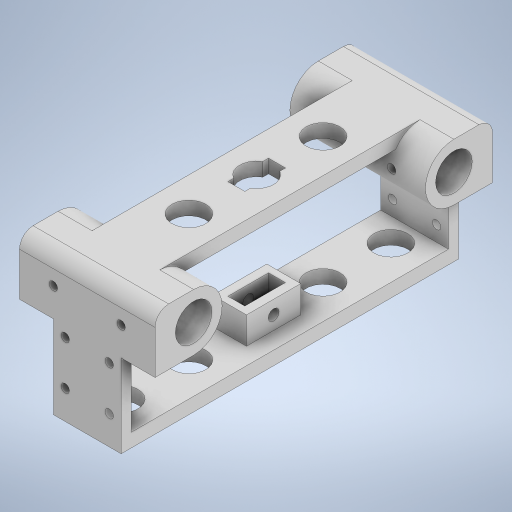
# Autodesk Inventor part: top
Saved by Autodesk Inventor 2024 (Build 280153000, 153)
## iProperties
Created: 2024-07-02
Part Number: top
Material: 일반
Document SubType Name: Modeling
Designer: Gihyeok Na
Density: 1 g/cm^3
Appearance: 기본값
Author: Gihyeok Na
Autodesk Inventor part; units mm, degrees
ref_plane "YZ Plane" through (0, 0, 0) normal (1, 0, 0) x (0, 1, 0)
ref_plane "XZ Plane" through (0, 0, 0) normal (0, 1, 0) x (-1, 0, 0)
ref_plane "XY Plane" through (0, 0, 0) normal (0, 0, 1) x (1, 0, 0)
sketch "스케치1" plane through (0, 0, 0) normal (1, 0, 0) x (0, 1, 0)
  line L0 (-15, -8.4) -> (15, -8.4)
  line L1 (15, -8.4) -> (15, -11.4)
  line L2 (15, -11.4) -> (-15, -11.4)
  line L3 (-15, -11.4) -> (-15, -8.4)
  line L4 (-15, -8.4) -> (15, -11.4) construction
  line L5 (15, -8.4) -> (-15, -11.4) construction
  line L6 (-10.7716, 0) -> (20.6854, 0) construction
  circle A0 centre (17.9, 0) radius 5.4
  circle A1 centre (17.9, 0) radius 8.4
  line L7 (9.5, -4.3302) -> (9.5, -23.7251) construction
  line L8 (15, -8.4) -> (17.9, -8.4)
  line L9 (9.5, 0) -> (9.5, -8.4)
  line L10 (56.0253, 38.4) -> (-49.003, 38.4) construction
  line L11 (-15, 85.2) -> (15, 85.2)
  line L12 (15, 85.2) -> (15, 88.2)
  line L13 (15, 88.2) -> (-15, 88.2)
  line L14 (-15, 88.2) -> (-15, 85.2)
  line L15 (-15, 85.2) -> (15, 88.2) construction
  line L16 (15, 85.2) -> (-15, 88.2) construction
  line L17 (-10.7716, 76.8) -> (20.6854, 76.8) construction
  circle A2 centre (17.9, 76.8) radius 5.4
  circle A3 centre (17.9, 76.8) radius 8.4
  line L18 (9.5, 81.1302) -> (9.5, 100.5251) construction
  line L19 (15, 85.2) -> (17.9, 85.2)
  line L20 (9.5, 76.8) -> (9.5, 85.2)
  line L21 (15, -11.4) -> (26.3, -11.4)
  line L22 (26.3, -11.4) -> (26.3, 0)
  line L23 (15, 88.2) -> (26.3, 88.2)
  line L24 (26.3, 88.2) -> (26.3, 76.8)
  point P0 (0, -9.9)
  point P1 (6.5, -8.4)
  point P2 (22.1201, -7.263)
  point P3 (0, 86.7)
  point P4 (6.5, 85.2)
  point P5 (22.1201, 84.063)
  dimension "d2" = 30
  dimension "d3" = 3
  dimension "d9" = 10.8
  dimension "d10" = 16.8
  dimension "d11" = 8.5
  dimension "d12" = 3
  dimension "d20" = 38.4
  constraints: 50 end point, 18 symmetric about line, 11 point on line, 7 point on circle, 4 centre point, 4 horizontal, 4 midpoint, 3 tangent, 2 coincident, 2 parallel, 1 perpendicular, 1 vertical, 2 other
  measures "d2" distance of L0.start L0.end
  measures "d3" distance of L0.end L1.end
  measures "d9" diameter of A0
  measures "d10" diameter of A1
  measures "d11" distance from line of point (6.5, -8.4) L1
  measures "d12" distance from line of L7 point (6.5, -8.4)
  measures "d20" distance from line of L10 A0.centre
extrude "돌출1" add sketch "스케치1" along normal mid plane 20
fillet "모깎기1" radius 4 2 edges at (0, 26.3, -11.4) (0, 26.3, 88.2)
sketch "스케치4" plane through (10, -15, -11.4) normal (0, 0, -1) x (-1, 0, 0)
  line L0 (-6.6272, 15) -> (50.9826, 15) construction
  line L1 (10, 54.1091) -> (10, -11.8144) construction
  circle A0 centre (3.5, 8.5) radius 1.25
  line L2 (20, 0) -> (0, 0) projected
  line L3 (0, 0) -> (0, 37.3) projected
  circle A1 centre (16.5, 8.5) radius 1.25
  circle A2 centre (3.5, 21.5) radius 1.25
  circle A3 centre (16.5, 21.5) radius 1.25
  circle A4 centre (10, 32.9) radius 1.25
  line L4 (20, 41.3) -> (0, 41.3) projected
  point P0 (10, 15)
  dimension "d22" = 2.5
  dimension "d23" = 8.5
  dimension "d24" = 3.5
  dimension "d27" = 2.5
  dimension "d28" = 8.4
  constraints: 5 centre point, 4 end point, 3 symmetric about line, 1 horizontal, 1 point on line, 1 vertical, 3 other
  measures "d22" diameter of A0
  measures "d23" distance from line of L2 A0.centre
  measures "d24" distance from line of L3 A0.centre
  measures "d27" diameter of A4
  measures "d28" distance from line of A4.centre L4
extrude "돌출4" cut sketch "스케치4" against normal through all contours A0 | A1 | A2 | A3
sketch "스케치5" plane through (-10, 0, 0) normal (-1, 0, 0) x (0, 0, 1)
  circle A0 centre (0, 17.9) radius 5.4 projected
  arc A1 (-7.4, 26.3) -> (-11.4, 22.3) centre (-7.4, 22.3) ccw projected
  line L0 (-11.4, 22.3) -> (-11.4, -15) projected
  line L1 (-11.4, -15) -> (-8.4, -15) projected
  line L2 (-8.4, -15) -> (-8.4, 9.5) projected
  line L3 (-8.4, 9.5) -> (0, 9.5) projected
  arc A2 (0, 9.5) -> (0, 26.3) centre (0, 17.9) ccw projected
  line L4 (0, 26.3) -> (-7.4, 26.3) projected
  circle A3 centre (76.8, 17.9) radius 5.4 projected
  arc A4 (88.2, 22.3) -> (84.2, 26.3) centre (84.2, 22.3) ccw projected
  line L5 (84.2, 26.3) -> (76.8, 26.3) projected
  arc A5 (76.8, 26.3) -> (76.8, 9.5) centre (76.8, 17.9) ccw projected
  line L6 (76.8, 9.5) -> (85.2, 9.5) projected
  line L7 (85.2, 9.5) -> (85.2, -15) projected
  line L8 (85.2, -15) -> (88.2, -15) projected
  line L9 (88.2, -15) -> (88.2, 22.3) projected
  line L10 (-8.4, -15) -> (85.2, -15)
  line L11 (-8.4, -11) -> (85.2, -11)
  line L12 (85.2, -15) -> (88.2, -15) projected
  line L13 (-8.4, 9.5) -> (-8.4, -15) projected
  line L14 (0, 26.3) -> (76.8, 26.3)
  circle A6 centre (0, 17.9) radius 5.4 projected
  circle A7 centre (76.8, 17.9) radius 5.4 projected
  line L15 (7.1554, 22.3) -> (69.6446, 22.3)
  point P0 (0, 0)
  point P1 (0, -6.5)
  point P2 (0, 6.5)
  point P3 (0, 0)
  point P4 (85.2, -4.062)
  dimension "d29" = 4
  dimension "d31" = 8.5
  dimension "d32" = 13
  dimension "d35" = 4
  constraints: 8 end point, 3 horizontal, 3 point on line, 2 point on circle, 2 tangent, 1 collinear, 1 perpendicular
  measures "d29" distance between parallel lines of L10 L11
  measures "d31" distance from line of L10 point (0, -6.5)
  measures "d32" distance of point (0, -6.5) point (0, 6.5)
  measures "d35" distance between parallel lines of L15 L14
extrude "돌출5" add sketch "스케치5" against normal up to surface (20 mm away) contours L14 A5 L15 A2 | L2 L11 L7 L10
sketch "스케치6" plane through (-10, -15, -11.4) normal (0, -1, 0) x (1, 0, 0)
  circle A0 centre (10, 10) radius 5
  line L0 (0, 0) -> (20, 0) projected
  line L1 (10, 10) -> (10, 54.4458) construction
  circle A1 centre (10, 89.6) radius 5
  line L2 (0, 99.6) -> (20, 99.6) projected
  circle A2 centre (10, 30) radius 5
  circle A3 centre (10, 69.6) radius 5
  circle A4 centre (10, 49.6) radius 5
  line L3 (7.5, 55.6) -> (7.5, 43.6)
  line L4 (7.5, 43.6) -> (12.5, 43.6)
  line L5 (12.5, 43.6) -> (12.5, 55.6)
  line L6 (12.5, 55.6) -> (7.5, 55.6)
  line L7 (7.5, 55.6) -> (12.5, 43.6) construction
  line L8 (7.5, 43.6) -> (12.5, 55.6) construction
  line L9 (5, 57.6) -> (5, 41.6)
  line L10 (5, 41.6) -> (15, 41.6)
  line L11 (15, 41.6) -> (15, 57.6)
  line L12 (15, 57.6) -> (5, 57.6)
  line L13 (5, 57.6) -> (15, 41.6) construction
  line L14 (5, 41.6) -> (15, 57.6) construction
  line L15 (20, 55.6) -> (0, 55.6)
  line L16 (0, 96.6) -> (0, 3) projected
  line L17 (20, 43.6) -> (0, 43.6)
  line L18 (20, 99.6) -> (20, 0) projected
  line L19 (0, 0) -> (0, 99.6) projected
  point P0 (10, 11.4)
  point P1 (7.5, 53.9301)
  point P2 (12.5, 53.9301)
  point P3 (12.5, 45.2699)
  point P4 (7.5, 45.2699)
  dimension "d38" = 10
  dimension "d39" = 10
  dimension "d40" = 10
  dimension "d41" = 10
  dimension "d44" = 20
  dimension "d51" = 20
  dimension "d94" = 12
  dimension "d95" = 5
  dimension "d96" = 16
  constraints: 30 end point, 5 centre point, 5 parallel, 4 midpoint, 4 point on line, 3 vertical, 2 perpendicular, 1 horizontal, 6 other
  measures "d38" diameter of A0
  measures "d39" distance from line of L1.start L0
  measures "d40" diameter of A1
  measures "d41" distance from line of L2 A1.centre
  measures "d44" distance of L1.start A2.centre
  measures "d51" distance of A1.centre A3.centre
  measures "d94" distance of L3.start L3.end
  measures "d95" distance of L4.end L3.end
  measures "d96" distance of L9.start L9.end
extrude "돌출6" cut sketch "스케치6" against normal up to surface (4 mm away) contours A0 | A4 L5 | A4 L3 | L5 A4 L3 | A1 | A2 | A3
extrude "돌출7" cut sketch "스케치6" against normal through all contours A4 L5 | A4 L3 | L5 A4 L3 | A2 | A3
sketch "스케치7" plane through (-10, 0, 0) normal (-1, 0, 0) x (0, 0, 1)
  arc A0 (0, 9.5) -> (7.1554, 22.3) centre (0, 17.9) ccw projected
  arc A1 (69.6446, 22.3) -> (76.8, 9.5) centre (76.8, 17.9) ccw projected
  line L0 (-8.4, 9.5) -> (0, 9.5) projected
  line L1 (-11.4, 22.3) -> (-11.4, -15) projected
  arc A2 (-7.4, 26.3) -> (-11.4, 22.3) centre (-7.4, 22.3) ccw projected
  line L2 (84.2, 26.3) -> (-7.4, 26.3) projected
  arc A3 (88.2, 22.3) -> (84.2, 26.3) centre (84.2, 22.3) ccw projected
  line L3 (88.2, -15) -> (88.2, 22.3) projected
  line L4 (76.8, 9.5) -> (85.2, 9.5) projected
  line L5 (-8.4, 9.5) -> (-11.4, 9.5)
  line L6 (85.2, 9.5) -> (88.2, 9.5)
  arc A4 (7.1554, 22.3) -> (0, 26.3) centre (0, 17.9) ccw
  line L7 (7.1554, 22.3) -> (69.6446, 22.3) projected
  arc A5 (76.8, 26.3) -> (69.6446, 22.3) centre (76.8, 17.9) ccw
  circle A6 centre (0, 17.9) radius 5.4 projected
  circle A7 centre (76.8, 17.9) radius 5.4 projected
  point P0 (0, 0)
  constraints: 5 point on line, 4 end point, 4 point on circle, 2 centre point, 2 coincident, 1 horizontal
extrude "돌출8" add sketch "스케치7" along normal blind 10 contours L0 L5 L1 A2 L2 A4 A0 | A5 L2 A3 L3 L6 L4 A1
sketch "스케치8" plane through (10, 0, 0) normal (1, 0, 0) x (0, 0, -1)
  line L0 (0, 9.5) -> (8.4, 9.5) projected
  arc A0 (-7.1554, 22.3) -> (0, 9.5) centre (0, 17.9) ccw projected
  arc A1 (0, 26.3) -> (-7.1554, 22.3) centre (0, 17.9) ccw projected
  line L1 (7.4, 26.3) -> (-84.2, 26.3) projected
  arc A2 (11.4, 22.3) -> (7.4, 26.3) centre (7.4, 22.3) ccw projected
  line L2 (11.4, -15) -> (11.4, 22.3) projected
  circle A3 centre (0, 17.9) radius 5.4 projected
  line L3 (8.4, 9.5) -> (11.4, 9.5) projected
  arc A4 (-76.8, 9.5) -> (-69.6446, 22.3) centre (-76.8, 17.9) ccw projected
  line L4 (-85.2, 9.5) -> (-76.8, 9.5) projected
  arc A5 (-69.6446, 22.3) -> (-76.8, 26.3) centre (-76.8, 17.9) ccw projected
  arc A6 (-84.2, 26.3) -> (-88.2, 22.3) centre (-84.2, 22.3) ccw projected
  circle A7 centre (-76.8, 17.9) radius 5.4 projected
  line L5 (-88.2, 9.5) -> (-85.2, 9.5) projected
  line L6 (-88.2, 22.3) -> (-88.2, -15) projected
  point P0 (0, 0)
extrude "돌출9" add sketch "스케치8" along normal blind 10
sketch "스케치9" plane through (10, -15, -11.4) normal (0, 0, -1) x (-1, 0, 0)
  circle A0 centre (16.5, 8.5) radius 1.25 projected
  circle A1 centre (3.5, 8.5) radius 1.25 projected
  circle A2 centre (3.5, 21.5) radius 1.25 projected
  circle A3 centre (16.5, 21.5) radius 1.25 projected
  line L0 (-10, 37.3) -> (30, 37.3) projected
  line L1 (-10, 24.5) -> (-10, 37.3) projected
  line L2 (0, 24.5) -> (-10, 24.5) projected
  line L3 (0, 0) -> (0, 24.5) projected
  line L4 (20, 0) -> (0, 0) projected
  line L5 (20, 24.5) -> (20, 0) projected
  line L6 (20, 24.5) -> (30, 24.5) projected
  line L7 (30, 37.3) -> (30, 24.5) projected
  line L8 (5, 37.3) -> (5, 41.3) projected
  line L9 (5, 37.3) -> (5, 41.3) projected
  line L10 (5, 37.3) -> (5, 41.3) projected
  line L11 (30, 41.3) -> (-10, 41.3) projected
  line L12 (-10, 37.3) -> (30, 37.3) projected
  line L13 (30, 41.3) -> (30, 37.3) projected
  line L14 (30, 41.3) -> (-10, 41.3) projected
  line L15 (-10, 37.3) -> (-10, 41.3) projected
  line L16 (-10, 32.9) -> (30, 32.9) construction
  circle A4 centre (-5, 32.9) radius 1.25
  circle A5 centre (25, 32.9) radius 1.25
  point P0 (10, 15)
  dimension "d64" = 8.4
  dimension "d65" = 2.5
  dimension "d66" = 2.5
  dimension "d67" = 5
  dimension "d68" = 5
  constraints: 4 point on line, 2 centre point, 2 end point, 1 perpendicular
  measures "d64" distance between parallel lines of L16 L11
  measures "d65" diameter of A4
  measures "d66" diameter of A5
  measures "d67" distance from line of L1 A4.centre
  measures "d68" distance from line of A5.centre L7
sketch "스케치10" plane through (10, -15, -11.4) normal (0, 0, -1) x (-1, 0, 0)
  circle A0 centre (16.5, 8.5) radius 1.25 projected
  circle A1 centre (3.5, 8.5) radius 1.25 projected
  circle A2 centre (3.5, 21.5) radius 1.25 projected
  circle A3 centre (16.5, 21.5) radius 1.25 projected
  line L0 (-10, 37.3) -> (30, 37.3) projected
  line L1 (-10, 24.5) -> (-10, 37.3) projected
  line L2 (0, 24.5) -> (-10, 24.5) projected
  line L3 (0, 0) -> (0, 24.5) projected
  line L4 (20, 0) -> (0, 0) projected
  line L5 (20, 24.5) -> (20, 0) projected
  line L6 (20, 24.5) -> (30, 24.5) projected
  line L7 (30, 37.3) -> (30, 24.5) projected
  line L8 (-10, 38.3) -> (30, 38.3) projected
  line L9 (-10, 37.3) -> (30, 37.3) projected
  line L10 (30, 41.3) -> (30, 37.3) projected
  line L11 (30, 41.3) -> (-10, 41.3) projected
  line L12 (-10, 37.3) -> (-10, 41.3) projected
  line L13 (10, 0) -> (10, 41.3) construction
  line L14 (5, 41.3) -> (15, 41.3) projected
  circle A4 centre (0, 32.9) radius 1.25
  circle A5 centre (20, 32.9) radius 1.25
  point P0 (10, 15)
  dimension "d69" = 2.5
  dimension "d70" = 8.4
  dimension "d71" = 10
  constraints: 2 centre point, 2 end point, 2 midpoint, 1 symmetric about line, 1 other
  measures "d69" diameter of A4
  measures "d70" distance from line of L11 A4.centre
  measures "d71" distance from line of A4.centre L13
extrude "돌출10" cut sketch "스케치10" along normal through all both and the other way through all contours A4 | A5
sketch "스케치11" plane through (-10, -11, 85.2) normal (0, 1, 0) x (1, 0, 0)
  point P0 (10, 85.2)
extrude "돌출16" cut sketch "스케치6" against normal through all contours L4 L3 A4 L5 | A4 L3 L6 L5
extrude "돌출17" add sketch "스케치6" against normal blind 12 contours L17 L5 A4 L11 | L11 L10 L9 L17 L4 | L9 A4 L3 L17 | A4 L5 | A4 L5 L15 L11 | L15 L6 L9 L12 L11 | L15 L3 A4 L9 | A4 L3
sketch "스케치15" plane through (5, -11, 30.2) normal (1, 0, 0) x (0, 0, -1)
  circle A0 centre (-8, 4) radius 1.6
  line L0 (0, 0) -> (-16, 0) projected
  line L1 (0, 0) -> (0, 8) projected
  line L2 (-16, 8) -> (0, 8) projected
  line L3 (-16, 0) -> (-16, 8) projected
  point P0 (30.2, 11)
  dimension "d101" = 3.2
  dimension "d102" = 4
  dimension "d103" = 8
  constraints: 1 centre point
  measures "d101" diameter of A0
  measures "d102" distance from line of L2 A0.centre
  measures "d103" distance from line of L1 A0.centre
extrude "돌출18" cut sketch "스케치15" along normal through all both and the other way through all contours A0
